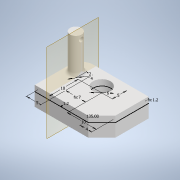
# Autodesk Inventor part: stringHold
Saved by Autodesk Inventor 2022 (Build 260153000, 153)
## iProperties
Created: 2021-07-01
Part Number: stringHold
Material: Generic
Document SubType Name: Modeling
Designer: dsdan
Density: 1 g/cm^3
Appearance: Default
Author: dsdan
Autodesk Inventor part; units mm, degrees
ref_plane "YZ Plane" through (0, 0, 0) normal (1, 0, 0) x (0, 1, 0)
ref_plane "XZ Plane" through (0, 0, 0) normal (0, 1, 0) x (-1, 0, 0)
ref_plane "XY Plane" through (0, 0, 0) normal (0, 0, 1) x (1, 0, 0)
sketch "Sketch1" plane through (0, 0, 0) normal (0, 1, 0) x (-1, 0, 0)
  circle A0 centre (0, 0) radius 3
  line L0 (12, 10) -> (-6, 10)
  line L1 (-10, 6) -> (-10, -5)
  line L2 (12, 10) -> (12, -1)
  line L3 (-10, -5) -> (8, -5)
  arc A1 (8, -5) -> (12, -1) centre (8, -1) ccw
  line L4 (-6, 10) -> (-10, 6)
  line L5 (-6, 10) -> (-0.3431, 10) construction
  line L6 (-6.4971, 11.2) -> (12, 11.2)
  line L7 (12, 11.2) -> (12, 10)
  line L8 (-10, -5) -> (-11.2, -5)
  line L9 (-11.2, -5) -> (-11.2, 6.4971)
  line L10 (-11.2, 6.4971) -> (-6.4971, 11.2)
  line L11 (12, 10) -> (12, 10)
  line L12 (-10, -5) -> (-10, -5)
  circle A2 centre (9, 0) radius 2
  point P0 (7, 0)
  dimension "d0" = 6
  dimension "d1" = 10
  dimension "d2" = 10
  dimension "d3" = 5
  dimension "d4" = 7
  dimension "d5" = 5
  dimension "d6" = 135
  dimension "d7" = 4
  dimension "d8" = 1.2
  dimension "d9" = 1.2
  dimension "d14" = 4
  dimension "d20" = 2
  constraints: 26 end point, 4 horizontal, 3 centre point, 3 perpendicular, 2 collinear, 2 horizontal alignment, 2 point on circle, 2 tangent, 1 coincident, 1 equal length, 1 vertical, 1 other
  measures "d0" diameter of A0
  measures "d1" distance from line of A0.centre L1
  measures "d2" distance from line of A0.centre L0
  measures "d3" distance from line of A0.centre L3
  measures "d4" distance of point (7, 0) A0.centre
  measures "d5" distance from line of point (7, 0) L2
  measures "d6" angle of L4 L5
  measures "d7" horizontal distance of L0.end L1.start
  measures "d8" distance between parallel lines of L0 L6
  measures "d9" distance between parallel lines of L1 L9
  measures "d14" diameter of A2
  measures "d20" distance of point (7, 0) A2.centre
extrude "Extrusion1" add sketch "Sketch1" along normal blind 2 contours L2 A1 L3 L1 L4 L0 | L0 L4 L1 L8 L9 L10 L6 L7 | A2
extrude "Extrusion2" add sketch "Sketch1" against normal blind 4.6 contours L0 L4 L1 L8 L9 L10 L6 L7
extrude "Extrusion3" add sketch "Sketch1" along normal blind 14 contours A2
sketch "Sketch4" plane through (0, 0, 0) normal (0, -1, 0) x (1, 0, 0)
  circle A0 centre (0, 0) radius 3 projected
  circle A1 centre (0, 0) radius 5.3
  circle A2 centre (0, 0) radius 3 projected
  line L0 (10, -5) -> (-8, -5) projected
  point P0 (-1.7578, -5)
  point P1 (1.7578, -5)
  dimension "d23" = 10.6
  constraints: 1 centre point, 1 coincident
  measures "d23" diameter of A1
extrude "Extrusion5" add sketch "Sketch4" along normal blind 4.6 contours A1 L0 picked at (-0.1205, -4.326)
ref_plane "Work Plane1" through (-7, 0, 0) normal (1, 0, 0) x (0, 1, 0)
sketch "Sketch5" plane through (-7, 0, 0) normal (1, 0, 0) x (0, 1, 0)
  circle A0 centre (12.5, 0) radius 0.75
  line L0 (2, 6.4971) -> (2, -5) projected
  point P0 (0, 0)
  dimension "d24" = 1.5
  dimension "d25" = 10.5
  constraints: 1 centre point
  measures "d24" diameter of A0
  measures "d25" distance from line of L0 A0.centre
extrude "Extrusion6" cut sketch "Sketch5" against normal through all
fillet "Fillet1" radius 1 1 edges at (-7, 2, 0)
equation "\"d4\" = -lensDistFromMetal + sensorDistFromLens - d1"
equation "\"d9\" = d8"
equation "\"sensorDistFromLens\" = 29"
equation "\"lensDistFromMetal\" = 12"
body "Solid1"
